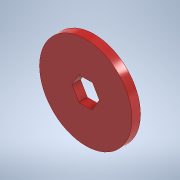
# Autodesk Inventor part: 1_2x2x3_16-hexBearing
Saved by Autodesk Inventor 2021.2 (Build 252289000, 289)
## iProperties
Created: 2020-11-08
Part Number: 1_2x2x3_16-hexBearing
Material: PC/ABS Plastic
Document SubType Name: Modeling
Designer: robst
Density: 0.357273 g/cm^3
Appearance: Red
Author: robst
Autodesk Inventor part; units mm, degrees
ref_plane "YZ Plane" through (0, 0, 0) normal (1, 0, 0) x (0, 1, 0)
ref_plane "XZ Plane" through (0, 0, 0) normal (0, 1, 0) x (-1, 0, 0)
ref_plane "XY Plane" through (0, 0, 0) normal (0, 0, 1) x (1, 0, 0)
sketch "Sketch1" plane through (0, 0, 0) normal (0, 0, 1) x (1, 0, 0)
  line L0 (3.6662, 6.35) -> (7.3323, 0)
  line L1 (7.3323, 0) -> (3.6662, -6.35)
  line L2 (3.6662, -6.35) -> (-3.6662, -6.35)
  line L3 (-3.6662, -6.35) -> (-7.3323, 0)
  line L4 (-7.3323, 0) -> (-3.6662, 6.35)
  line L5 (-3.6662, 6.35) -> (3.6662, 6.35)
  circle A0 centre (0, 0) radius 25.273
  circle A1 centre (0, 0) radius 7.3323 construction
  dimension "d0" = 12.7
  dimension "d2" = 50.546
  dimension "d3" = 17.9407
  constraints: 12 end point, 3 coincident, 1 centre point, 1 horizontal, 1 horizontal alignment, 15 other
  measures "d0" distance between parallel lines of L2 L5
  measures "d2" diameter of A0
extrude "Extrusion1" add sketch "Sketch1" against normal blind 4.7625
thicken "Reduce Outside Diameter" operation add thickness 0.127 both sides no extend neighbours yes toward (-0.9967573, 0.0804666, 0) faces at (25.191, -2.0336, -3.175)
thicken "Thicken2" operation add thickness 0.127 both sides no extend neighbours yes toward (-0.8660254, -0.5, 0) faces at (-4.8882, -4.2333, -1.5875) (-6.1103, 2.1167, -1.5875) (-1.2221, 6.35, -1.5875) (4.8882, 4.2333, -1.5875) (11.0881, 6.012, 0) (1.2221, -6.35, -1.5875)
equation "\"d0\" = hexSize"
equation "\"d2\" = externalDiameter - 2 * printSpacing"
equation "\"d4\" = thickness"
equation "\"d6\" = printSpacing"
equation "\"d7\" = printSpacing"
equation "\"d8\" = printSpacing"
equation "\"d9\" = printSpacing"
equation "\"hexSize\" = 12.7"
equation "\"externalDiameter\" = 50.8"
equation "\"thickness\" = 4.7625"
equation "\"printSpacing\" = 0.127"
body "Solid1"
